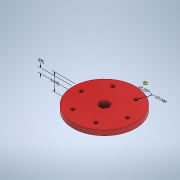
# Autodesk Inventor part: attachementToTripod
Saved by Autodesk Inventor 2022 (Build 260153000, 153)
## iProperties
Created: 2021-02-15
Part Number: attachementToTripod
Material: PC/ABS Plastic
Document SubType Name: Modeling
Designer: robst
Density: 0.357273 g/cm^3
Appearance: Red
Author: robst
Autodesk Inventor part; units mm, degrees
ref_plane "YZ Plane" through (0, 0, 0) normal (1, 0, 0) x (0, 1, 0)
ref_plane "XZ Plane" through (0, 0, 0) normal (0, 1, 0) x (-1, 0, 0)
ref_plane "XY Plane" through (0, 0, 0) normal (0, 0, 1) x (1, 0, 0)
sketch "Sketch2" plane through (0, 0, 0) normal (0, 0, 1) x (1, 0, 0)
  line L0 (-60.325, 0) -> (-60.325, -9.525)
  line L1 (-60.325, -9.525) -> (-12.7, -9.525)
  line L2 (-10.795, -44.525) -> (0, -44.525)
  line L3 (-60.325, 0) -> (0, 0)
  line L4 (0, 0) -> (0, -44.525) construction
  line L5 (0, 0) -> (0, -44.525)
  line L6 (0, -53.43) -> (0, 8.905) projected
  line L7 (-12.7, -9.525) -> (-10.795, -44.525)
  dimension "d0" = 60.325
  dimension "d3" = 9.525
  dimension "d4" = 35
  dimension "d64" = 10.795
  constraints: 14 end point, 3 vertical, 2 horizontal, 1 perpendicular
  measures "d0" distance from line of L0 L3.end
  measures "d3" distance from line of L1 L3.end
  measures "d4" distance from line of L2.start L1
  measures "d64" horizontal distance of L2.start L3.end
revolve "Revolution1" add sketch "Sketch2" angle 360 about axis through (0, -10, 0) along (0, 1, 0)
sketch "Sketch5" plane through (0, -9.525, 0) normal (0, -1, 0) x (1, 0, 0)
  circle A0 centre (0, 0) radius 34.925 construction
  line L0 (30.2767, -23.2881) -> (30.3048, -23.2474)
  spline S0 degree 2 poles (30.3048, -23.2474) (30.4192, -23.1689) (30.7643, -22.822) (30.8732, -22.6645) knots 0 0 0 1 2 2 2
  spline S1 degree 2 poles (30.8732, -22.6645) (31.2175, -22.1669) (31.0657, -21.4311) (30.4766, -21.0236) knots 0 0 0 1 2 2 2
  line L1 (30.4766, -21.0236) -> (30.3192, -20.9147)
  line L2 (30.3192, -20.9147) -> (29.4128, -22.2249)
  line L3 (29.4128, -22.2249) -> (28.7577, -21.7717)
  line L4 (28.7577, -21.7717) -> (29.6465, -20.4869)
  line L5 (29.6465, -20.4869) -> (25.5991, -17.6869)
  line L6 (25.5991, -17.6869) -> (26.1472, -16.8947)
  line L7 (26.1472, -16.8947) -> (30.1946, -19.6947)
  line L8 (30.1946, -19.6947) -> (30.5635, -19.1615)
  line L9 (30.5635, -19.1615) -> (31.2186, -19.6147)
  line L10 (31.2186, -19.6147) -> (30.8497, -20.1479)
  line L11 (30.8497, -20.1479) -> (31.0071, -20.2568)
  spline S2 degree 2 poles (31.0071, -20.2568) (31.8501, -20.84) (32.1681, -22.2689) (31.6411, -23.0306) knots 0 0 0 1 2 2 2
  spline S3 degree 2 poles (31.6411, -23.0306) (31.4901, -23.249) (31.1528, -23.6389) (31.0029, -23.7904) knots 0 0 0 1 2 2 2
  line L12 (31.0029, -23.7904) -> (30.2767, -23.2881)
  line L13 (23.4719, -20.4315) -> (24.0931, -19.6952)
  line L14 (24.0931, -19.6952) -> (28.4636, -23.3822)
  line L15 (28.4636, -23.3822) -> (27.8425, -24.1185)
  line L16 (27.8425, -24.1185) -> (23.4719, -20.4315)
  line L17 (28.5256, -24.7836) -> (29.2303, -23.9482)
  line L18 (29.2303, -23.9482) -> (29.9949, -24.5933)
  line L19 (29.9949, -24.5933) -> (29.2902, -25.4287)
  line L20 (29.2902, -25.4287) -> (28.5256, -24.7836)
  line L21 (21.8315, -22.1757) -> (22.5074, -21.4893)
  line L22 (22.5074, -21.4893) -> (28.1787, -27.0744)
  line L23 (28.1787, -27.0744) -> (27.5027, -27.7607)
  line L24 (27.5027, -27.7607) -> (21.8315, -22.1757)
  spline S4 degree 2 poles (18.8163, -24.6214) (19.8941, -23.7743) (22.0288, -24.0519) (22.9065, -25.1685) knots 0 0 0 1 2 2 2
  spline S5 degree 2 poles (22.9065, -25.1685) (23.769, -26.2657) (23.6412, -28.4712) (22.7139, -29.2001) knots 0 0 0 1 2 2 2
  spline S6 degree 2 poles (22.7139, -29.2001) (22.2964, -29.5282) (21.4599, -29.7931) (21.0198, -29.7227) knots 0 0 0 1 2 2 2
  spline S7 degree 2 poles (21.0198, -29.7227) (20.5748, -29.6563) (19.7336, -29.1157) (19.31, -28.5769) knots 0 0 0 1 2 2 2
  line L25 (19.31, -28.5769) -> (18.9857, -28.1642)
  line L26 (18.9857, -28.1642) -> (22.0975, -25.7181)
  spline S8 degree 2 poles (22.0975, -25.7181) (21.4831, -24.9365) (20.0441, -24.7245) (19.345, -25.2741) knots 0 0 0 1 2 2 2
  spline S9 degree 2 poles (19.345, -25.2741) (19.0974, -25.4687) (18.7046, -25.9581) (18.5791, -26.1982) knots 0 0 0 1 2 2 2
  spline S10 degree 2 poles (18.5791, -26.1982) (18.4515, -26.4555) (18.3035, -26.8468) (18.2723, -26.997) knots 0 0 0 1 2 2 2
  line L27 (18.2723, -26.997) -> (18.2286, -27.0313)
  line L28 (18.2286, -27.0313) -> (17.5799, -26.206)
  spline S11 degree 2 poles (17.5799, -26.206) (17.669, -26.0496) (17.945, -25.5813) (18.066, -25.4155) knots 0 0 0 1 2 2 2
  spline S12 degree 2 poles (18.066, -25.4155) (18.2348, -25.1807) (18.5444, -24.8352) (18.8163, -24.6214) knots 0 0 0 1 2 2 2
  spline S13 degree 2 poles (20.1777, -28.1619) (20.4278, -28.4601) (20.9051, -28.8075) (21.1448, -28.8626) knots 0 0 0 1 2 2 2
  spline S14 degree 2 poles (21.1448, -28.8626) (21.4094, -28.9295) (21.9633, -28.7847) (22.2691, -28.5443) knots 0 0 0 1 2 2 2
  spline S15 degree 2 poles (22.2691, -28.5443) (22.5701, -28.3077) (22.8513, -27.7961) (22.8887, -27.4839) knots 0 0 0 1 2 2 2
  spline S16 degree 2 poles (22.8887, -27.4839) (22.9174, -27.1707) (22.7525, -26.6013) (22.5516, -26.2958) knots 0 0 0 1 2 2 2
  line L29 (22.5516, -26.2958) -> (20.1777, -28.1619)
  line L30 (16.9957, -31.0317) -> (18.0577, -30.426)
  line L31 (18.0577, -30.426) -> (18.7797, -31.6918)
  line L32 (18.7797, -31.6918) -> (17.7177, -32.2976)
  line L33 (17.7177, -32.2976) -> (16.9957, -31.0317)
  line L34 (14.8847, -27.3306) -> (15.9467, -26.7249)
  line L35 (15.9467, -26.7249) -> (16.6687, -27.9907)
  line L36 (16.6687, -27.9907) -> (15.6067, -28.5965)
  line L37 (15.6067, -28.5965) -> (14.8847, -27.3306)
  spline S17 degree 2 poles (7.233, -30.9053) (7.3235, -30.7911) (7.6238, -30.3894) (7.7783, -30.2514) knots 0 0 0 1 2 2 2
  spline S18 degree 2 poles (7.7783, -30.2514) (7.9869, -30.0538) (8.4084, -29.792) (8.8255, -29.6785) knots 0 0 0 1 2 2 2
  spline S19 degree 2 poles (8.8255, -29.6785) (9.1652, -29.5861) (9.8486, -29.6754) (10.1442, -29.8446) knots 0 0 0 1 2 2 2
  spline S20 degree 2 poles (10.1442, -29.8446) (10.4262, -30.011) (10.8759, -30.6054) (10.9764, -30.9748) knots 0 0 0 1 2 2 2
  spline S21 degree 2 poles (10.9764, -30.9748) (11.132, -31.5469) (10.8698, -32.4885) (10.4087, -32.8635) knots 0 0 0 1 2 2 2
  spline S22 degree 2 poles (10.4087, -32.8635) (10.0023, -33.2045) (8.7828, -33.709) (8.0613, -33.9501) knots 0 0 0 1 2 2 2
  line L38 (8.0613, -33.9501) -> (8.1099, -34.1288)
  spline S23 degree 2 poles (8.1099, -34.1288) (8.1974, -34.4506) (8.5027, -34.7963) (8.7122, -34.8609) knots 0 0 0 1 2 2 2
  spline S24 degree 2 poles (8.7122, -34.8609) (8.9218, -34.9255) (9.4537, -34.8576) (9.7278, -34.783) knots 0 0 0 1 2 2 2
  spline S25 degree 2 poles (9.7278, -34.783) (10.0495, -34.6955) (10.8676, -34.2682) (11.2523, -33.9651) knots 0 0 0 1 2 2 2
  line L39 (11.2523, -33.9651) -> (11.3059, -33.9505)
  line L40 (11.3059, -33.9505) -> (11.5637, -34.8979)
  spline S26 degree 2 poles (11.5637, -34.8979) (11.3269, -35.0391) (10.4162, -35.4789) (9.9455, -35.6069) knots 0 0 0 1 2 2 2
  spline S27 degree 2 poles (9.9455, -35.6069) (9.3735, -35.7625) (8.5443, -35.7961) (8.1712, -35.648) knots 0 0 0 1 2 2 2
  spline S28 degree 2 poles (8.1712, -35.648) (7.8057, -35.5043) (7.3117, -34.8643) (7.1707, -34.3459) knots 0 0 0 1 2 2 2
  line L41 (7.1707, -34.3459) -> (6.1446, -30.5742)
  line L42 (6.1446, -30.5742) -> (7.0742, -30.3213)
  line L43 (7.0742, -30.3213) -> (7.233, -30.9053)
  line L44 (7.4437, -31.6799) -> (7.8603, -33.2112)
  spline S29 degree 2 poles (7.8603, -33.2112) (8.1859, -33.0906) (9.1653, -32.7154) (9.4552, -32.5342) knots 0 0 0 1 2 2 2
  spline S30 degree 2 poles (9.4552, -32.5342) (9.7938, -32.3205) (10.1484, -31.7184) (10.0349, -31.3014) knots 0 0 0 1 2 2 2
  spline S31 degree 2 poles (10.0349, -31.3014) (9.9052, -30.8247) (9.2377, -30.4879) (8.7253, -30.6273) knots 0 0 0 1 2 2 2
  spline S32 degree 2 poles (8.7253, -30.6273) (8.2903, -30.7456) (7.6774, -31.3155) (7.4437, -31.6799) knots 0 0 0 1 2 2 2
  spline S33 degree 2 poles (3.0779, -30.858) (3.8564, -30.7633) (4.8411, -31.5454) (4.9582, -32.5078) knots 0 0 0 1 2 2 2
  line L45 (4.9582, -32.5078) -> (5.341, -35.6524)
  line L46 (5.341, -35.6524) -> (5.9846, -35.574)
  line L47 (5.9846, -35.574) -> (6.0809, -36.3648)
  line L48 (6.0809, -36.3648) -> (5.4372, -36.4431)
  line L49 (5.4372, -36.4431) -> (5.6357, -38.0737)
  line L50 (5.6357, -38.0737) -> (4.6794, -38.19)
  line L51 (4.6794, -38.19) -> (4.481, -36.5595)
  line L52 (4.481, -36.5595) -> (2.7217, -36.7736)
  line L53 (2.7217, -36.7736) -> (2.6255, -35.9829)
  line L54 (2.6255, -35.9829) -> (4.3847, -35.7688)
  line L55 (4.3847, -35.7688) -> (4.0557, -33.0655)
  spline S34 degree 2 poles (4.0557, -33.0655) (4.0035, -32.6364) (3.9154, -32.1682) (3.7866, -31.9786) knots 0 0 0 1 2 2 2
  spline S35 degree 2 poles (3.7866, -31.9786) (3.6791, -31.8113) (3.2713, -31.6805) (2.9403, -31.7208) knots 0 0 0 1 2 2 2
  spline S36 degree 2 poles (2.9403, -31.7208) (2.7073, -31.7491) (2.2893, -31.9431) (2.1964, -31.9979) knots 0 0 0 1 2 2 2
  line L56 (2.1964, -31.9979) -> (2.1413, -32.0047)
  line L57 (2.1413, -32.0047) -> (2.0368, -31.1465)
  spline S37 degree 2 poles (2.0368, -31.1465) (2.2976, -31.0401) (2.8388, -30.8871) (3.0779, -30.858) knots 0 0 0 1 2 2 2
  spline S38 degree 2 poles (-0.4091, -31.0085) (0.3751, -31.0018) (1.2658, -31.8896) (1.274, -32.8591) knots 0 0 0 1 2 2 2
  line L58 (1.274, -32.8591) -> (1.301, -36.0267)
  line L59 (1.301, -36.0267) -> (1.9493, -36.0212)
  line L60 (1.9493, -36.0212) -> (1.9561, -36.8178)
  line L61 (1.9561, -36.8178) -> (1.3078, -36.8233)
  line L62 (1.3078, -36.8233) -> (1.3218, -38.4658)
  line L63 (1.3218, -38.4658) -> (0.3585, -38.474)
  line L64 (0.3585, -38.474) -> (0.3445, -36.8315)
  line L65 (0.3445, -36.8315) -> (-1.4277, -36.8466)
  line L66 (-1.4277, -36.8466) -> (-1.4344, -36.05)
  line L67 (-1.4344, -36.05) -> (0.3377, -36.0349)
  line L68 (0.3377, -36.0349) -> (0.3145, -33.3118)
  spline S39 degree 2 poles (0.3145, -33.3118) (0.3109, -32.8796) (0.2759, -32.4044) (0.1692, -32.2015) knots 0 0 0 1 2 2 2
  spline S40 degree 2 poles (0.1692, -32.2015) (0.0813, -32.0232) (-0.3093, -31.8474) (-0.6427, -31.8503) knots 0 0 0 1 2 2 2
  spline S41 degree 2 poles (-0.6427, -31.8503) (-0.8774, -31.8523) (-1.3146, -31.998) (-1.413, -32.0421) knots 0 0 0 1 2 2 2
  line L69 (-1.413, -32.0421) -> (-1.4686, -32.0426)
  line L70 (-1.4686, -32.0426) -> (-1.4759, -31.1781)
  spline S42 degree 2 poles (-1.4759, -31.1781) (-1.2049, -31.1017) (-0.6499, -31.0105) (-0.4091, -31.0085) knots 0 0 0 1 2 2 2
  spline S43 degree 2 poles (-5.4224, -31.2738) (-5.2945, -31.204) (-4.8611, -30.9517) (-4.665, -30.885) knots 0 0 0 1 2 2 2
  spline S44 degree 2 poles (-4.665, -30.885) (-4.3957, -30.7848) (-3.9054, -30.7085) (-3.4771, -30.7671) knots 0 0 0 1 2 2 2
  spline S45 degree 2 poles (-3.4771, -30.7671) (-3.1284, -30.8148) (-2.5342, -31.1641) (-2.3282, -31.4353) knots 0 0 0 1 2 2 2
  spline S46 degree 2 poles (-2.3282, -31.4353) (-2.1337, -31.6988) (-1.9521, -32.4217) (-2.004, -32.801) knots 0 0 0 1 2 2 2
  spline S47 degree 2 poles (-2.004, -32.801) (-2.0844, -33.3883) (-2.6938, -34.1526) (-3.2648, -34.3175) knots 0 0 0 1 2 2 2
  spline S48 degree 2 poles (-3.2648, -34.3175) (-3.7722, -34.4725) (-5.0918, -34.4602) (-5.8502, -34.4001) knots 0 0 0 1 2 2 2
  line L71 (-5.8502, -34.4001) -> (-5.8753, -34.5836)
  spline S49 degree 2 poles (-5.8753, -34.5836) (-5.9205, -34.914) (-5.7747, -35.3516) (-5.607, -35.4929) knots 0 0 0 1 2 2 2
  spline S50 degree 2 poles (-5.607, -35.4929) (-5.4394, -35.6343) (-4.9233, -35.7797) (-4.6418, -35.8182) knots 0 0 0 1 2 2 2
  spline S51 degree 2 poles (-4.6418, -35.8182) (-4.3115, -35.8634) (-3.3914, -35.7898) (-2.9189, -35.6612) knots 0 0 0 1 2 2 2
  line L72 (-2.9189, -35.6612) -> (-2.8638, -35.6688)
  line L73 (-2.8638, -35.6688) -> (-2.9969, -36.6415)
  spline S52 degree 2 poles (-2.9969, -36.6415) (-3.27, -36.679) (-4.2801, -36.7277) (-4.7635, -36.6616) knots 0 0 0 1 2 2 2
  spline S53 degree 2 poles (-4.7635, -36.6616) (-5.3508, -36.5813) (-6.1272, -36.2881) (-6.4127, -36.0059) knots 0 0 0 1 2 2 2
  spline S54 degree 2 poles (-6.4127, -36.0059) (-6.6929, -35.7308) (-6.8975, -34.9486) (-6.8247, -34.4164) knots 0 0 0 1 2 2 2
  line L74 (-6.8247, -34.4164) -> (-6.2948, -30.5436)
  line L75 (-6.2948, -30.5436) -> (-5.3404, -30.6742)
  line L76 (-5.3404, -30.6742) -> (-5.4224, -31.2738)
  line L77 (-5.5312, -32.0691) -> (-5.7464, -33.6415)
  spline S55 degree 2 poles (-5.7464, -33.6415) (-5.3996, -33.6577) (-4.3514, -33.6952) (-4.0137, -33.6417) knots 0 0 0 1 2 2 2
  spline S56 degree 2 poles (-4.0137, -33.6417) (-3.6185, -33.5773) (-3.0568, -33.1618) (-2.9982, -32.7335) knots 0 0 0 1 2 2 2
  spline S57 degree 2 poles (-2.9982, -32.7335) (-2.9313, -32.2441) (-3.4141, -31.6732) (-3.9402, -31.6012) knots 0 0 0 1 2 2 2
  spline S58 degree 2 poles (-3.9402, -31.6012) (-4.3869, -31.5401) (-5.1738, -31.8251) (-5.5312, -32.0691) knots 0 0 0 1 2 2 2
  spline S59 degree 2 poles (-9.7347, -29.4216) (-9.1687, -29.5978) (-8.3394, -30.2374) (-8.1135, -30.6957) knots 0 0 0 1 2 2 2
  spline S60 degree 2 poles (-8.1135, -30.6957) (-7.8856, -31.1482) (-7.8481, -32.3369) (-8.072, -33.0562) knots 0 0 0 1 2 2 2
  spline S61 degree 2 poles (-8.072, -33.0562) (-8.2958, -33.7755) (-9.0057, -34.7058) (-9.4401, -34.9586) knots 0 0 0 1 2 2 2
  spline S62 degree 2 poles (-9.4401, -34.9586) (-9.8763, -35.2174) (-10.9566, -35.3016) (-11.5108, -35.1291) knots 0 0 0 1 2 2 2
  spline S63 degree 2 poles (-11.5108, -35.1291) (-11.9589, -34.9896) (-12.7173, -34.4755) (-12.9902, -34.2095) knots 0 0 0 1 2 2 2
  line L78 (-12.9902, -34.2095) -> (-12.6691, -33.1777)
  line L79 (-12.6691, -33.1777) -> (-12.616, -33.1942)
  spline S64 degree 2 poles (-12.616, -33.1942) (-12.5415, -33.308) (-12.301, -33.6156) (-12.1177, -33.7956) knots 0 0 0 1 2 2 2
  spline S65 degree 2 poles (-12.1177, -33.7956) (-11.9524, -33.9504) (-11.4795, -34.2593) (-11.2436, -34.3327) knots 0 0 0 1 2 2 2
  spline S66 degree 2 poles (-11.2436, -34.3327) (-10.5302, -34.5547) (-9.3277, -33.7455) (-9.0212, -32.7608) knots 0 0 0 1 2 2 2
  spline S67 degree 2 poles (-9.0212, -32.7608) (-8.7222, -31.7997) (-9.2236, -30.4602) (-9.9666, -30.229) knots 0 0 0 1 2 2 2
  spline S68 degree 2 poles (-9.9666, -30.229) (-10.4147, -30.0895) (-11.3439, -30.2078) (-11.7463, -30.3995) knots 0 0 0 1 2 2 2
  line L80 (-11.7463, -30.3995) -> (-11.7994, -30.3829)
  line L81 (-11.7994, -30.3829) -> (-11.4783, -29.3511)
  spline S69 degree 2 poles (-11.4783, -29.3511) (-11.3225, -29.3285) (-10.8529, -29.2741) (-10.6749, -29.2842) knots 0 0 0 1 2 2 2
  spline S70 degree 2 poles (-10.6749, -29.2842) (-10.4171, -29.2869) (-10.0236, -29.3317) (-9.7347, -29.4216) knots 0 0 0 1 2 2 2
  line L82 (-16.1877, -26.669) -> (-15.3301, -27.1077)
  line L83 (-15.3301, -27.1077) -> (-16.8149, -30.0104)
  spline S71 degree 2 poles (-16.8149, -30.0104) (-16.9949, -30.3623) (-17.2383, -31.0007) (-17.2321, -31.2328) knots 0 0 0 1 2 2 2
  spline S72 degree 2 poles (-17.2321, -31.2328) (-17.2261, -31.4786) (-16.9479, -31.8568) (-16.629, -32.0199) knots 0 0 0 1 2 2 2
  spline S73 degree 2 poles (-16.629, -32.0199) (-16.3102, -32.183) (-15.4596, -32.188) (-14.9947, -32.0791) knots 0 0 0 1 2 2 2
  line L84 (-14.9947, -32.0791) -> (-13.0486, -28.2748)
  line L85 (-13.0486, -28.2748) -> (-12.191, -28.7135)
  line L86 (-12.191, -28.7135) -> (-15.8159, -35.7998)
  line L87 (-15.8159, -35.7998) -> (-16.6735, -35.3611)
  line L88 (-16.6735, -35.3611) -> (-15.363, -32.7992)
  spline S74 degree 2 poles (-15.363, -32.7992) (-15.925, -32.9487) (-16.8528, -32.9319) (-17.2706, -32.7182) knots 0 0 0 1 2 2 2
  spline S75 degree 2 poles (-17.2706, -32.7182) (-18.0183, -32.3357) (-18.3587, -30.9131) (-17.8778, -29.973) knots 0 0 0 1 2 2 2
  line L89 (-17.8778, -29.973) -> (-16.1877, -26.669)
  spline S76 degree 2 poles (-19.2059, -24.3188) (-18.1186, -25.1537) (-17.8599, -27.2908) (-18.7248, -28.4173) knots 0 0 0 1 2 2 2
  spline S77 degree 2 poles (-18.7248, -28.4173) (-19.5747, -29.5242) (-21.7434, -29.9456) (-22.6789, -29.2273) knots 0 0 0 1 2 2 2
  spline S78 degree 2 poles (-22.6789, -29.2273) (-23.1001, -28.9039) (-23.5635, -28.1588) (-23.6041, -27.7149) knots 0 0 0 1 2 2 2
  spline S79 degree 2 poles (-23.6041, -27.7149) (-23.6497, -27.2673) (-23.3339, -26.3186) (-22.9165, -25.775) knots 0 0 0 1 2 2 2
  line L90 (-22.9165, -25.775) -> (-22.5968, -25.3587)
  line L91 (-22.5968, -25.3587) -> (-19.4573, -27.7693)
  spline S80 degree 2 poles (-19.4573, -27.7693) (-18.8519, -26.9807) (-19.0022, -25.534) (-19.7075, -24.9924) knots 0 0 0 1 2 2 2
  spline S81 degree 2 poles (-19.7075, -24.9924) (-19.9573, -24.8006) (-20.5287, -24.541) (-20.7923, -24.4787) knots 0 0 0 1 2 2 2
  spline S82 degree 2 poles (-20.7923, -24.4787) (-21.0732, -24.4187) (-21.4889, -24.372) (-21.6421, -24.3789) knots 0 0 0 1 2 2 2
  line L92 (-21.6421, -24.3789) -> (-21.6862, -24.3451)
  line L93 (-21.6862, -24.3451) -> (-21.0469, -23.5125)
  spline S83 degree 2 poles (-21.0469, -23.5125) (-20.8733, -23.5601) (-20.3513, -23.7118) (-20.1608, -23.788) knots 0 0 0 1 2 2 2
  spline S84 degree 2 poles (-20.1608, -23.788) (-19.8915, -23.8936) (-19.4801, -24.1082) (-19.2059, -24.3188) knots 0 0 0 1 2 2 2
  spline S85 degree 2 poles (-22.2999, -26.5131) (-22.527, -26.8292) (-22.7456, -27.3776) (-22.7398, -27.6234) knots 0 0 0 1 2 2 2
  spline S86 degree 2 poles (-22.7398, -27.6234) (-22.7392, -27.8964) (-22.462, -28.3973) (-22.1534, -28.6342) knots 0 0 0 1 2 2 2
  spline S87 degree 2 poles (-22.1534, -28.6342) (-21.8498, -28.8674) (-21.2845, -29.0133) (-20.9728, -28.9724) knots 0 0 0 1 2 2 2
  spline S88 degree 2 poles (-20.9728, -28.9724) (-20.6622, -28.9228) (-20.1512, -28.6223) (-19.9048, -28.3521) knots 0 0 0 1 2 2 2
  line L94 (-19.9048, -28.3521) -> (-22.2999, -26.5131)
  line L95 (-25.8186, -17.5864) -> (-28.3773, -19.6859)
  spline S89 degree 2 poles (-28.3773, -19.6859) (-28.6828, -19.9366) (-29.164, -20.4113) (-29.2445, -20.6052) knots 0 0 0 1 2 2 2
  spline S90 degree 2 poles (-29.2445, -20.6052) (-29.3394, -20.8108) (-29.2532, -21.2274) (-29.0456, -21.4804) knots 0 0 0 1 2 2 2
  spline S91 degree 2 poles (-29.0456, -21.4804) (-28.8576, -21.7095) (-28.1451, -22.0035) (-27.6506, -22.061) knots 0 0 0 1 2 2 2
  spline S92 degree 2 poles (-27.6506, -22.061) (-27.5877, -22.0014) (-27.4093, -21.8391) (-27.2852, -21.7373) knots 0 0 0 1 2 2 2
  line L96 (-27.2852, -21.7373) -> (-24.3732, -19.3479)
  line L97 (-24.3732, -19.3479) -> (-23.7622, -20.0926)
  line L98 (-23.7622, -20.0926) -> (-26.3209, -22.1921)
  spline S93 degree 2 poles (-26.3209, -22.1921) (-26.6264, -22.4428) (-27.1076, -22.9175) (-27.1881, -23.1114) knots 0 0 0 1 2 2 2
  spline S94 degree 2 poles (-27.1881, -23.1114) (-27.283, -23.317) (-27.1968, -23.7336) (-26.9892, -23.9866) knots 0 0 0 1 2 2 2
  spline S95 degree 2 poles (-26.9892, -23.9866) (-26.7934, -24.2253) (-26.0578, -24.5084) (-25.6202, -24.5647) knots 0 0 0 1 2 2 2
  line L99 (-25.6202, -24.5647) -> (-22.3168, -21.8541)
  line L100 (-22.3168, -21.8541) -> (-21.7058, -22.5988)
  line L101 (-21.7058, -22.5988) -> (-26.1262, -26.2259)
  line L102 (-26.1262, -26.2259) -> (-26.7373, -25.4812)
  line L103 (-26.7373, -25.4812) -> (-26.2504, -25.0817)
  spline S96 degree 2 poles (-26.2504, -25.0817) (-26.7805, -25.0295) (-27.5704, -24.719) (-27.8524, -24.3753) knots 0 0 0 1 2 2 2
  spline S97 degree 2 poles (-27.8524, -24.3753) (-28.1736, -23.9839) (-28.313, -23.0839) (-28.0365, -22.5934) knots 0 0 0 1 2 2 2
  spline S98 degree 2 poles (-28.0365, -22.5934) (-28.6917, -22.5639) (-29.6033, -22.2415) (-29.9088, -21.8691) knots 0 0 0 1 2 2 2
  spline S99 degree 2 poles (-29.9088, -21.8691) (-30.1438, -21.5827) (-30.3511, -20.97) (-30.2916, -20.6336) knots 0 0 0 1 2 2 2
  spline S100 degree 2 poles (-30.2916, -20.6336) (-30.236, -20.2924) (-29.7951, -19.6032) (-29.3416, -19.2311) knots 0 0 0 1 2 2 2
  line L104 (-29.3416, -19.2311) -> (-26.4296, -16.8417)
  line L105 (-26.4296, -16.8417) -> (-25.8186, -17.5864)
  spline S101 degree 2 poles (-27.9752, -13.3288) (-27.3687, -14.5582) (-28.0811, -16.5897) (-29.3548, -17.218) knots 0 0 0 1 2 2 2
  spline S102 degree 2 poles (-29.3548, -17.218) (-30.6063, -17.8354) (-32.7379, -17.2551) (-33.2597, -16.1974) knots 0 0 0 1 2 2 2
  spline S103 degree 2 poles (-33.2597, -16.1974) (-33.4947, -15.7211) (-33.5811, -14.848) (-33.4215, -14.4318) knots 0 0 0 1 2 2 2
  spline S104 degree 2 poles (-33.4215, -14.4318) (-33.2646, -14.0102) (-32.5621, -13.2987) (-31.9474, -12.9954) knots 0 0 0 1 2 2 2
  line L106 (-31.9474, -12.9954) -> (-31.4766, -12.7632)
  line L107 (-31.4766, -12.7632) -> (-29.7255, -16.313)
  spline S105 degree 2 poles (-29.7255, -16.313) (-28.8339, -15.8732) (-28.3295, -14.5089) (-28.7229, -13.7114) knots 0 0 0 1 2 2 2
  spline S106 degree 2 poles (-28.7229, -13.7114) (-28.8622, -13.429) (-29.26, -12.9436) (-29.469, -12.7712) knots 0 0 0 1 2 2 2
  spline S107 degree 2 poles (-29.469, -12.7712) (-29.6945, -12.5933) (-30.0468, -12.3677) (-30.1873, -12.3062) knots 0 0 0 1 2 2 2
  line L108 (-30.1873, -12.3062) -> (-30.2119, -12.2564)
  line L109 (-30.2119, -12.2564) -> (-29.2704, -11.7919)
  spline S108 degree 2 poles (-29.2704, -11.7919) (-29.1358, -11.9114) (-28.7345, -12.2781) (-28.5973, -12.4307) knots 0 0 0 1 2 2 2
  spline S109 degree 2 poles (-28.5973, -12.4307) (-28.4023, -12.6444) (-28.1282, -13.0187) (-27.9752, -13.3288) knots 0 0 0 1 2 2 2
  spline S110 degree 2 poles (-31.7204, -13.9301) (-32.0638, -14.1133) (-32.5023, -14.5086) (-32.6057, -14.7317) knots 0 0 0 1 2 2 2
  spline S111 degree 2 poles (-32.6057, -14.7317) (-32.7257, -14.9769) (-32.6984, -15.5486) (-32.5263, -15.8975) knots 0 0 0 1 2 2 2
  spline S112 degree 2 poles (-32.5263, -15.8975) (-32.3569, -16.2409) (-31.9143, -16.6216) (-31.6166, -16.7226) knots 0 0 0 1 2 2 2
  spline S113 degree 2 poles (-31.6166, -16.7226) (-31.3161, -16.8154) (-30.7249, -16.7716) (-30.3845, -16.6381) knots 0 0 0 1 2 2 2
  line L110 (-30.3845, -16.6381) -> (-31.7204, -13.9301)
  line L111 (-30.553, -6.308) -> (-30.2903, -7.2347)
  line L112 (-30.2903, -7.2347) -> (-33.427, -8.1242)
  spline S114 degree 2 poles (-33.427, -8.1242) (-33.8072, -8.232) (-34.4405, -8.4886) (-34.6062, -8.6511) knots 0 0 0 1 2 2 2
  spline S115 degree 2 poles (-34.6062, -8.6511) (-34.7821, -8.8229) (-34.8696, -9.2842) (-34.7719, -9.6288) knots 0 0 0 1 2 2 2
  spline S116 degree 2 poles (-34.7719, -9.6288) (-34.6742, -9.9733) (-34.0986, -10.5996) (-33.7022, -10.8659) knots 0 0 0 1 2 2 2
  line L113 (-33.7022, -10.8659) -> (-29.5912, -9.7002)
  line L114 (-29.5912, -9.7002) -> (-29.3284, -10.6269)
  line L115 (-29.3284, -10.6269) -> (-34.8296, -12.1868)
  line L116 (-34.8296, -12.1868) -> (-35.0924, -11.2601)
  line L117 (-35.0924, -11.2601) -> (-34.4805, -11.0866)
  spline S117 degree 2 poles (-34.4805, -11.0866) (-34.9727, -10.7768) (-35.5922, -10.086) (-35.7202, -9.6345) knots 0 0 0 1 2 2 2
  spline S118 degree 2 poles (-35.7202, -9.6345) (-35.9493, -8.8265) (-35.1394, -7.6084) (-34.1235, -7.3204) knots 0 0 0 1 2 2 2
  line L118 (-34.1235, -7.3204) -> (-30.553, -6.308)
  spline S119 degree 2 poles (-30.8413, -3.2409) (-30.7425, -4.0189) (-31.5194, -5.0077) (-32.4811, -5.13) knots 0 0 0 1 2 2 2
  line L119 (-32.4811, -5.13) -> (-35.6237, -5.5293)
  line L120 (-35.6237, -5.5293) -> (-35.5419, -6.1725)
  line L121 (-35.5419, -6.1725) -> (-36.3321, -6.273)
  line L122 (-36.3321, -6.273) -> (-36.4139, -5.6297)
  line L123 (-36.4139, -5.6297) -> (-38.0433, -5.8368)
  line L124 (-38.0433, -5.8368) -> (-38.1648, -4.8812)
  line L125 (-38.1648, -4.8812) -> (-36.5353, -4.6741)
  line L126 (-36.5353, -4.6741) -> (-36.7587, -2.916)
  line L127 (-36.7587, -2.916) -> (-35.9685, -2.8156)
  line L128 (-35.9685, -2.8156) -> (-35.7451, -4.5737)
  line L129 (-35.7451, -4.5737) -> (-33.0436, -4.2304)
  spline S120 degree 2 poles (-33.0436, -4.2304) (-32.6148, -4.1759) (-32.147, -4.0853) (-31.9581, -3.9555) knots 0 0 0 1 2 2 2
  spline S121 degree 2 poles (-31.9581, -3.9555) (-31.7914, -3.8472) (-31.6628, -3.4387) (-31.7048, -3.1079) knots 0 0 0 1 2 2 2
  spline S122 degree 2 poles (-31.7048, -3.1079) (-31.7344, -2.8751) (-31.9306, -2.4581) (-31.9859, -2.3655) knots 0 0 0 1 2 2 2
  line L130 (-31.9859, -2.3655) -> (-31.9929, -2.3104)
  line L131 (-31.9929, -2.3104) -> (-31.1353, -2.2014)
  spline S123 degree 2 poles (-31.1353, -2.2014) (-31.0275, -2.4616) (-30.8717, -3.002) (-30.8413, -3.2409) knots 0 0 0 1 2 2 2
  line L132 (-31.1171, 0.3593) -> (-37.833, 0.5475)
  line L133 (-37.833, 0.5475) -> (-37.9046, -2.0079)
  line L134 (-37.9046, -2.0079) -> (-38.8058, -1.9827)
  line L135 (-38.8058, -1.9827) -> (-38.6342, 4.1405)
  line L136 (-38.6342, 4.1405) -> (-37.733, 4.1153)
  line L137 (-37.733, 4.1153) -> (-37.8046, 1.5598)
  line L138 (-37.8046, 1.5598) -> (-31.0888, 1.3716)
  line L139 (-31.0888, 1.3716) -> (-31.1171, 0.3593)
  spline S124 degree 2 poles (-32.6248, 9.8171) (-31.2139, 9.5056) (-29.9758, 7.8094) (-30.226, 6.6758) knots 0 0 0 1 2 2 2
  spline S125 degree 2 poles (-30.226, 6.6758) (-30.4829, 5.512) (-32.363, 4.5295) (-33.7257, 4.8304) knots 0 0 0 1 2 2 2
  spline S126 degree 2 poles (-33.7257, 4.8304) (-35.1246, 5.1392) (-36.3708, 6.8561) (-36.1232, 7.9777) knots 0 0 0 1 2 2 2
  spline S127 degree 2 poles (-36.1232, 7.9777) (-35.873, 9.1113) (-34.0298, 10.1272) (-32.6248, 9.8171) knots 0 0 0 1 2 2 2
  spline S128 degree 2 poles (-32.8392, 8.8463) (-33.9245, 9.0859) (-35.1541, 8.5289) (-35.3152, 7.7993) knots 0 0 0 1 2 2 2
  spline S129 degree 2 poles (-35.3152, 7.7993) (-35.4763, 7.0697) (-34.5968, 6.0408) (-33.5114, 5.8012) knots 0 0 0 1 2 2 2
  spline S130 degree 2 poles (-33.5114, 5.8012) (-32.4562, 5.5682) (-31.1951, 6.1246) (-31.034, 6.8542) knots 0 0 0 1 2 2 2
  spline S131 degree 2 poles (-31.034, 6.8542) (-30.8743, 7.5778) (-31.7658, 8.6093) (-32.8392, 8.8463) knots 0 0 0 1 2 2 2
  line L140 (-28.7817, 11.8329) -> (-34.9526, 14.4895)
  line L141 (-34.9526, 14.4895) -> (-35.9635, 12.1414)
  line L142 (-35.9635, 12.1414) -> (-36.7916, 12.4979)
  line L143 (-36.7916, 12.4979) -> (-34.3694, 18.1243)
  line L144 (-34.3694, 18.1243) -> (-33.5413, 17.7678)
  line L145 (-33.5413, 17.7678) -> (-34.5522, 15.4197)
  line L146 (-34.5522, 15.4197) -> (-28.3813, 12.763)
  line L147 (-28.3813, 12.763) -> (-28.7817, 11.8329)
  line L148 (-29.2463, 20.7319) -> (-29.2728, 20.6902)
  spline S132 degree 2 poles (-29.2728, 20.6902) (-29.3584, 20.6129) (-29.4978, 20.4161) (-29.5871, 20.2754) knots 0 0 0 1 2 2 2
  spline S133 degree 2 poles (-29.5871, 20.2754) (-29.7955, 19.9469) (-29.9189, 19.1183) (-29.8225, 18.6477) knots 0 0 0 1 2 2 2
  line L149 (-29.8225, 18.6477) -> (-26.3967, 16.4745)
  line L150 (-26.3967, 16.4745) -> (-26.9127, 15.6611)
  line L151 (-26.9127, 15.6611) -> (-31.7412, 18.7241)
  line L152 (-31.7412, 18.7241) -> (-31.2252, 19.5375)
  line L153 (-31.2252, 19.5375) -> (-30.5056, 19.081)
  spline S134 degree 2 poles (-30.5056, 19.081) (-30.6208, 19.7757) (-30.524, 20.643) (-30.3255, 20.9558) knots 0 0 0 1 2 2 2
  spline S135 degree 2 poles (-30.3255, 20.9558) (-30.2461, 21.081) (-30.1563, 21.1995) (-30.091, 21.2678) knots 0 0 0 1 2 2 2
  line L154 (-30.091, 21.2678) -> (-29.2463, 20.7319)
  line L155 (-24.1987, 19.5652) -> (-24.7927, 18.8069)
  line L156 (-24.7927, 18.8069) -> (-29.2943, 22.3327)
  line L157 (-29.2943, 22.3327) -> (-28.7003, 23.0911)
  line L158 (-28.7003, 23.0911) -> (-24.1987, 19.5652)
  line L159 (-29.4071, 23.731) -> (-30.081, 22.8705)
  line L160 (-30.081, 22.8705) -> (-30.8686, 23.4873)
  line L161 (-30.8686, 23.4873) -> (-30.1946, 24.3478)
  line L162 (-30.1946, 24.3478) -> (-29.4071, 23.731)
  spline S136 degree 2 poles (-22.0291, 26.1953) (-21.0266, 25.1719) (-20.8175, 23.0083) (-21.563, 22.278) knots 0 0 0 1 2 2 2
  spline S137 degree 2 poles (-21.563, 22.278) (-21.8674, 21.9799) (-22.4733, 21.663) (-22.8585, 21.5709) knots 0 0 0 1 2 2 2
  line L163 (-22.8585, 21.5709) -> (-21.1819, 19.8593)
  line L164 (-21.1819, 19.8593) -> (-21.8701, 19.1852)
  line L165 (-21.8701, 19.1852) -> (-27.3449, 24.7743)
  line L166 (-27.3449, 24.7743) -> (-26.6567, 25.4484)
  line L167 (-26.6567, 25.4484) -> (-26.2375, 25.0205)
  spline S138 degree 2 poles (-26.2375, 25.0205) (-26.2107, 25.505) (-25.8868, 26.4273) (-25.5206, 26.786) knots 0 0 0 1 2 2 2
  spline S139 degree 2 poles (-25.5206, 26.786) (-24.8192, 27.473) (-22.9451, 27.1305) (-22.0291, 26.1953) knots 0 0 0 1 2 2 2
  spline S140 degree 2 poles (-22.6615, 25.4202) (-23.3485, 26.1216) (-24.5503, 26.4572) (-25.0488, 25.9689) knots 0 0 0 1 2 2 2
  spline S141 degree 2 poles (-25.0488, 25.9689) (-25.3399, 25.6837) (-25.632, 24.8876) (-25.6758, 24.4471) knots 0 0 0 1 2 2 2
  line L168 (-25.6758, 24.4471) -> (-23.4029, 22.1267)
  spline S142 degree 2 poles (-23.4029, 22.1267) (-23.0085, 22.2624) (-22.5297, 22.5413) (-22.2826, 22.7832) knots 0 0 0 1 2 2 2
  spline S143 degree 2 poles (-22.2826, 22.7832) (-21.7489, 23.3061) (-21.9269, 24.6703) (-22.6615, 25.4202) knots 0 0 0 1 2 2 2
  spline S144 degree 2 poles (-16.8133, 29.6322) (-16.008, 28.4324) (-16.2841, 26.3507) (-17.2481, 25.7037) knots 0 0 0 1 2 2 2
  spline S145 degree 2 poles (-17.2481, 25.7037) (-18.2376, 25.0396) (-20.2758, 25.6275) (-21.0535, 26.7863) knots 0 0 0 1 2 2 2
  spline S146 degree 2 poles (-21.0535, 26.7863) (-21.8519, 27.9758) (-21.5673, 30.0781) (-20.6136, 30.7182) knots 0 0 0 1 2 2 2
  spline S147 degree 2 poles (-20.6136, 30.7182) (-19.6497, 31.3652) (-17.6151, 30.8269) (-16.8133, 29.6322) knots 0 0 0 1 2 2 2
  spline S148 degree 2 poles (-17.6388, 29.0782) (-18.2582, 30.0011) (-19.5321, 30.4475) (-20.1525, 30.0311) knots 0 0 0 1 2 2 2
  spline S149 degree 2 poles (-20.1525, 30.0311) (-20.7729, 29.6147) (-20.8475, 28.2632) (-20.228, 27.3403) knots 0 0 0 1 2 2 2
  spline S150 degree 2 poles (-20.228, 27.3403) (-19.6258, 26.4431) (-18.3296, 25.9744) (-17.7092, 26.3908) knots 0 0 0 1 2 2 2
  spline S151 degree 2 poles (-17.7092, 26.3908) (-17.0939, 26.8038) (-17.0262, 28.1655) (-17.6388, 29.0782) knots 0 0 0 1 2 2 2
  line L169 (-10.3034, 29.4417) -> (-11.1879, 29.0603)
  line L170 (-11.1879, 29.0603) -> (-11.4178, 29.5933)
  spline S152 degree 2 poles (-11.4178, 29.5933) (-11.5486, 29.3351) (-11.7513, 28.9787) (-11.9138, 28.7943) knots 0 0 0 1 2 2 2
  spline S153 degree 2 poles (-11.9138, 28.7943) (-12.0618, 28.6228) (-12.4228, 28.3528) (-12.6893, 28.2379) knots 0 0 0 1 2 2 2
  spline S154 degree 2 poles (-12.6893, 28.2379) (-13.1203, 28.052) (-14.0001, 28.0963) (-14.4044, 28.3321) knots 0 0 0 1 2 2 2
  spline S155 degree 2 poles (-14.4044, 28.3321) (-14.8088, 28.5679) (-15.5325, 29.4663) (-15.8186, 30.1297) knots 0 0 0 1 2 2 2
  spline S156 degree 2 poles (-15.8186, 30.1297) (-16.1169, 30.8215) (-16.195, 31.9848) (-16.0469, 32.4992) knots 0 0 0 1 2 2 2
  spline S157 degree 2 poles (-16.0469, 32.4992) (-15.9045, 32.9642) (-15.2624, 33.7051) (-14.8144, 33.8983) knots 0 0 0 1 2 2 2
  spline S158 degree 2 poles (-14.8144, 33.8983) (-14.4232, 34.067) (-13.7634, 34.1431) (-13.3619, 34.1011) knots 0 0 0 1 2 2 2
  line L171 (-13.3619, 34.1011) -> (-14.3401, 36.3691)
  line L172 (-14.3401, 36.3691) -> (-13.4555, 36.7506)
  line L173 (-13.4555, 36.7506) -> (-10.3034, 29.4417)
  line L174 (-11.7382, 30.336) -> (-13.0465, 33.3696)
  spline S159 degree 2 poles (-13.0465, 33.3696) (-13.4438, 33.3865) (-14.0168, 33.2806) (-14.3173, 33.151) knots 0 0 0 1 2 2 2
  spline S160 degree 2 poles (-14.3173, 33.151) (-14.9977, 32.8576) (-15.3287, 31.5044) (-14.913, 30.5404) knots 0 0 0 1 2 2 2
  spline S161 degree 2 poles (-14.913, 30.5404) (-14.512, 29.6105) (-13.4992, 28.8839) (-12.8471, 29.1651) knots 0 0 0 1 2 2 2
  spline S162 degree 2 poles (-12.8471, 29.1651) (-12.5012, 29.3143) (-11.9351, 29.9351) (-11.7382, 30.336) knots 0 0 0 1 2 2 2
  line L175 (-7.517, 30.1994) -> (-8.6975, 29.8811)
  line L176 (-8.6975, 29.8811) -> (-9.077, 31.2881)
  line L177 (-9.077, 31.2881) -> (-7.8965, 31.6064)
  line L178 (-7.8965, 31.6064) -> (-7.517, 30.1994)
  line L179 (-4.9112, 30.7287) -> (-5.8599, 30.562)
  line L180 (-5.8599, 30.562) -> (-6.8496, 36.1938)
  line L181 (-6.8496, 36.1938) -> (-5.9009, 36.3605)
  line L182 (-5.9009, 36.3605) -> (-4.9112, 30.7287)
  line L183 (-5.9986, 37.3089) -> (-7.0751, 37.1197)
  line L184 (-7.0751, 37.1197) -> (-7.2482, 38.105)
  line L185 (-7.2482, 38.105) -> (-6.1717, 38.2941)
  line L186 (-6.1717, 38.2941) -> (-5.9986, 37.3089)
  spline S163 degree 2 poles (1.1354, 34.208) (1.1965, 32.7767) (-0.0948, 31.028) (-1.1374, 30.9835) knots 0 0 0 1 2 2 2
  spline S164 degree 2 poles (-1.1374, 30.9835) (-1.5631, 30.9654) (-2.2255, 31.1349) (-2.5735, 31.324) knots 0 0 0 1 2 2 2
  line L187 (-2.5735, 31.324) -> (-2.4713, 28.9302)
  line L188 (-2.4713, 28.9302) -> (-3.4337, 28.8891)
  line L189 (-3.4337, 28.8891) -> (-3.7675, 36.7058)
  line L190 (-3.7675, 36.7058) -> (-2.8051, 36.7469)
  line L191 (-2.8051, 36.7469) -> (-2.7795, 36.1484)
  spline S165 degree 2 poles (-2.7795, 36.1484) (-2.4356, 36.4907) (-1.578, 36.96) (-1.066, 36.9818) knots 0 0 0 1 2 2 2
  spline S166 degree 2 poles (-1.066, 36.9818) (-0.085, 37.0237) (1.0795, 35.5159) (1.1354, 34.208) knots 0 0 0 1 2 2 2
  spline S167 degree 2 poles (0.1468, 34.0545) (0.1049, 35.0355) (-0.5643, 36.0885) (-1.2614, 36.0587) knots 0 0 0 1 2 2 2
  spline S168 degree 2 poles (-1.2614, 36.0587) (-1.6686, 36.0414) (-2.4181, 35.6447) (-2.7453, 35.3464) knots 0 0 0 1 2 2 2
  line L192 (-2.7453, 35.3464) -> (-2.6067, 32.1013)
  spline S169 degree 2 poles (-2.6067, 32.1013) (-2.2227, 31.9385) (-1.6802, 31.8257) (-1.3347, 31.8404) knots 0 0 0 1 2 2 2
  spline S170 degree 2 poles (-1.3347, 31.8404) (-0.5882, 31.8723) (0.1916, 33.0057) (0.1468, 34.0545) knots 0 0 0 1 2 2 2
  spline S171 degree 2 poles (3.9632, 30.7569) (3.1834, 30.8402) (2.4005, 31.8243) (2.5035, 32.7883) knots 0 0 0 1 2 2 2
  line L193 (2.5035, 32.7883) -> (2.84, 35.9382)
  line L194 (2.84, 35.9382) -> (2.1953, 36.0071)
  line L195 (2.1953, 36.0071) -> (2.28, 36.7991)
  line L196 (2.28, 36.7991) -> (2.9247, 36.7302)
  line L197 (2.9247, 36.7302) -> (3.0992, 38.3635)
  line L198 (3.0992, 38.3635) -> (4.057, 38.2612)
  line L199 (4.057, 38.2612) -> (3.8825, 36.6279)
  line L200 (3.8825, 36.6279) -> (5.6447, 36.4396)
  line L201 (5.6447, 36.4396) -> (5.5601, 35.6475)
  line L202 (5.5601, 35.6475) -> (3.7979, 35.8358)
  line L203 (3.7979, 35.8358) -> (3.5086, 33.1281)
  spline S172 degree 2 poles (3.5086, 33.1281) (3.4627, 32.6982) (3.4428, 32.2222) (3.5256, 32.0084) knots 0 0 0 1 2 2 2
  spline S173 degree 2 poles (3.5256, 32.0084) (3.5925, 31.8212) (3.9603, 31.6018) (4.2919, 31.5663) knots 0 0 0 1 2 2 2
  spline S174 degree 2 poles (4.2919, 31.5663) (4.5252, 31.5414) (4.9762, 31.636) (5.0791, 31.6685) knots 0 0 0 1 2 2 2
  line L204 (5.0791, 31.6685) -> (5.1343, 31.6626)
  line L205 (5.1343, 31.6626) -> (5.0425, 30.803)
  spline S175 degree 2 poles (5.0425, 30.803) (4.7644, 30.7582) (4.2026, 30.7313) (3.9632, 30.7569) knots 0 0 0 1 2 2 2
  spline S176 degree 2 poles (15.3764, 33.1447) (15.2022, 32.6824) (14.5592, 31.9745) (14.1556, 31.7966) knots 0 0 0 1 2 2 2
  spline S177 degree 2 poles (14.1556, 31.7966) (13.6486, 31.572) (12.5074, 31.5732) (11.7447, 31.8607) knots 0 0 0 1 2 2 2
  line L206 (11.7447, 31.8607) -> (10.9415, 32.1634)
  line L207 (10.9415, 32.1634) -> (9.9397, 29.5054)
  line L208 (9.9397, 29.5054) -> (8.992, 29.8626)
  line L209 (8.992, 29.8626) -> (11.6795, 36.9929)
  line L210 (11.6795, 36.9929) -> (13.4708, 36.3178)
  spline S178 degree 2 poles (13.4708, 36.3178) (14.1064, 36.0782) (14.9178, 35.5348) (15.1695, 35.1694) knots 0 0 0 1 2 2 2
  spline S179 degree 2 poles (15.1695, 35.1694) (15.4658, 34.7475) (15.6007, 33.7398) (15.3764, 33.1447) knots 0 0 0 1 2 2 2
  spline S180 degree 2 poles (14.3774, 33.4882) (14.5168, 33.858) (14.4673, 34.497) (14.2726, 34.7683) knots 0 0 0 1 2 2 2
  spline S181 degree 2 poles (14.2726, 34.7683) (14.1039, 35.0035) (13.5487, 35.3513) (13.1037, 35.519) knots 0 0 0 1 2 2 2
  line L211 (13.1037, 35.519) -> (12.3179, 35.8152)
  line L212 (12.3179, 35.8152) -> (11.2464, 32.9723)
  line L213 (11.2464, 32.9723) -> (11.8936, 32.7284)
  spline S182 degree 2 poles (11.8936, 32.7284) (12.4714, 32.5106) (13.2518, 32.4276) (13.5744, 32.5832) knots 0 0 0 1 2 2 2
  spline S183 degree 2 poles (13.5744, 32.5832) (13.8688, 32.7164) (14.2489, 33.1473) (14.3774, 33.4882) knots 0 0 0 1 2 2 2
  line L214 (23.0573, 31.2817) -> (16.8135, 26.1859)
  line L215 (16.8135, 26.1859) -> (15.8844, 26.7615)
  line L216 (15.8844, 26.7615) -> (17.6662, 34.6213)
  line L217 (17.6662, 34.6213) -> (18.5901, 34.049)
  line L218 (18.5901, 34.049) -> (17.0522, 27.5562)
  line L219 (17.0522, 27.5562) -> (22.1807, 31.8247)
  line L220 (22.1807, 31.8247) -> (23.0573, 31.2817)
  spline S184 degree 2 poles (25.5384, 23.9478) (24.1442, 22.4447) (21.9645, 21.8471) (21.0545, 22.6911) knots 0 0 0 1 2 2 2
  spline S185 degree 2 poles (21.0545, 22.6911) (20.1309, 23.5478) (20.5973, 25.785) (21.962, 27.2564) knots 0 0 0 1 2 2 2
  spline S186 degree 2 poles (21.962, 27.2564) (23.3646, 28.7686) (25.5359, 29.3571) (26.4504, 28.5089) knots 0 0 0 1 2 2 2
  spline S187 degree 2 poles (26.4504, 28.5089) (27.3695, 27.6565) (26.8905, 25.4056) (25.5384, 23.9478) knots 0 0 0 1 2 2 2
  spline S188 degree 2 poles (22.9996, 23.1357) (23.3645, 23.3111) (24.2445, 24.0783) (24.7778, 24.6533) knots 0 0 0 1 2 2 2
  spline S189 degree 2 poles (24.7778, 24.6533) (25.3111, 25.2282) (26.0058, 26.1589) (26.1571, 26.5491) knots 0 0 0 1 2 2 2
  spline S190 degree 2 poles (26.1571, 26.5491) (26.3085, 26.9393) (26.1875, 27.5989) (25.8752, 27.8886) knots 0 0 0 1 2 2 2
  spline S191 degree 2 poles (25.8752, 27.8886) (25.5628, 28.1784) (24.8869, 28.2578) (24.4962, 28.0727) knots 0 0 0 1 2 2 2
  spline S192 degree 2 poles (24.4962, 28.0727) (24.1185, 27.8925) (23.2307, 27.0988) (22.7226, 26.551) knots 0 0 0 1 2 2 2
  spline S193 degree 2 poles (22.7226, 26.551) (22.1767, 25.9624) (21.5185, 25.1074) (21.3507, 24.6904) knots 0 0 0 1 2 2 2
  spline S194 degree 2 poles (21.3507, 24.6904) (21.1906, 24.2999) (21.3038, 23.6137) (21.6298, 23.3114) knots 0 0 0 1 2 2 2
  spline S195 degree 2 poles (21.6298, 23.3114) (21.9376, 23.0258) (22.6135, 22.9464) (22.9996, 23.1357) knots 0 0 0 1 2 2 2
  spline S196 degree 2 poles (30.3482, 22.891) (30.1823, 23.1139) (29.7453, 23.4737) (29.5025, 23.6241) knots 0 0 0 1 2 2 2
  spline S197 degree 2 poles (29.5025, 23.6241) (29.2709, 23.7596) (28.875, 23.9191) (28.711, 23.9741) knots 0 0 0 1 2 2 2
  line L221 (28.711, 23.9741) -> (28.6741, 24.0236)
  line L222 (28.6741, 24.0236) -> (29.541, 24.6688)
  spline S198 degree 2 poles (29.541, 24.6688) (29.8838, 24.5081) (30.7986, 23.7649) (31.1046, 23.3537) knots 0 0 0 1 2 2 2
  spline S199 degree 2 poles (31.1046, 23.3537) (31.4142, 22.9376) (31.7066, 22.193) (31.7163, 21.8077) knots 0 0 0 1 2 2 2
  spline S200 degree 2 poles (31.7163, 21.8077) (31.7221, 21.3964) (31.3688, 20.7024) (30.9923, 20.4222) knots 0 0 0 1 2 2 2
  spline S201 degree 2 poles (30.9923, 20.4222) (30.487, 20.0462) (29.2301, 20.1424) (28.7845, 20.5343) knots 0 0 0 1 2 2 2
  line L223 (28.7845, 20.5343) -> (28.725, 20.4901)
  spline S202 degree 2 poles (28.725, 20.4901) (28.8292, 20.2674) (28.9789, 19.6938) (28.9406, 19.3728) knots 0 0 0 1 2 2 2
  spline S203 degree 2 poles (28.9406, 19.3728) (28.9073, 19.0555) (28.5294, 18.4049) (28.1282, 18.1063) knots 0 0 0 1 2 2 2
  spline S204 degree 2 poles (28.1282, 18.1063) (27.717, 17.8003) (26.8084, 17.5629) (26.3492, 17.6214) knots 0 0 0 1 2 2 2
  spline S205 degree 2 poles (26.3492, 17.6214) (25.8727, 17.6825) (25.0213, 18.2266) (24.6637, 18.7072) knots 0 0 0 1 2 2 2
  spline S206 degree 2 poles (24.6637, 18.7072) (24.3209, 19.1679) (23.8729, 20.2354) (23.7979, 20.6568) knots 0 0 0 1 2 2 2
  line L224 (23.7979, 20.6568) -> (24.6649, 21.3019)
  line L225 (24.6649, 21.3019) -> (24.7091, 21.2425)
  spline S207 degree 2 poles (24.7091, 21.2425) (24.7126, 20.8448) (25.0146, 19.7149) (25.3353, 19.2839) knots 0 0 0 1 2 2 2
  spline S208 degree 2 poles (25.3353, 19.2839) (25.5233, 19.0312) (26.0578, 18.6439) (26.3665, 18.6118) knots 0 0 0 1 2 2 2
  spline S209 degree 2 poles (26.3665, 18.6118) (26.6714, 18.5848) (27.2364, 18.7358) (27.5683, 18.9828) knots 0 0 0 1 2 2 2
  spline S210 degree 2 poles (27.5683, 18.9828) (27.9002, 19.2297) (28.1874, 19.7437) (28.1823, 20.0092) knots 0 0 0 1 2 2 2
  spline S211 degree 2 poles (28.1823, 20.0092) (28.1771, 20.2748) (27.921, 20.8154) (27.7146, 21.0928) knots 0 0 0 1 2 2 2
  line L226 (27.7146, 21.0928) -> (27.4565, 21.4396)
  line L227 (27.4565, 21.4396) -> (28.1352, 21.9447)
  line L228 (28.1352, 21.9447) -> (28.338, 21.6722)
  spline S212 degree 2 poles (28.338, 21.6722) (28.7472, 21.1223) (29.7884, 20.8195) (30.2887, 21.1918) knots 0 0 0 1 2 2 2
  spline S213 degree 2 poles (30.2887, 21.1918) (30.5216, 21.3651) (30.7208, 21.7904) (30.7129, 22.0078) knots 0 0 0 1 2 2 2
  spline S214 degree 2 poles (30.7129, 22.0078) (30.7027, 22.2388) (30.5067, 22.678) (30.3482, 22.891) knots 0 0 0 1 2 2 2
  dimension "d18" = 69.85
  constraints: 1 centre point, 1 coincident, 1 other
  measures "d18" diameter of A0
extrude "ExtrusionForText" cut sketch "Sketch5" against normal blind 1.27
sketch "Sketch13" plane through (0, -9.525, 0) normal (0, -1, 0) x (1, 0, 0)
  point P0 (0, 0)
  point P1 (44.45, 0)
  point P2 (22.225, 38.4948)
  point P3 (-22.225, 38.4948)
  point P4 (-44.45, 0)
  point P5 (-22.225, -38.4948)
  point P6 (22.225, -38.4948)
  dimension "d65" = 44.45
  dimension "d68" = 360
  constraints: 7 other
  measures "d65" distance of point (44.45, 0) point (0, 0)
hole "Hole6" at (44.45, -9.525, 0) at (22.225, -9.525, 38.4948) at (-22.225, -9.525, 38.4948) at (-44.45, -9.525, 0) at (-22.225, -9.525, -38.4948) at (22.225, -9.525, -38.4948) direction (0, 1, 0) diameter 6.3246 end through all counterbore diameter 6.5278 counterbore depth 6.1214
fillet "Fillet2" radius 1.27 1 edges at (10.795, -44.525, 0)
sketch "Sketch16" plane through (0, 0, 0) normal (0, 1, 0) x (1, 0, 0)
  point P0 (0, 0)
  point P1 (0, 0)
  constraints: 1 coincident
hole "Hole7" at (0, 0, 0) direction (0, -1, 0) diameter 11.9888 end through all clearance for "Flat Head Machine Screw" size "M10" standard "Ansi Metric M Profile"
sketch "Sketch18" plane through (0, 0, 0) normal (0, 1, 0) x (1, 0, 0)
  line L0 (9.9616, 0) -> (4.9808, -8.627)
  line L1 (4.9808, -8.627) -> (-4.9808, -8.627)
  line L2 (-4.9808, -8.627) -> (-9.9616, 0)
  line L3 (-9.9616, 0) -> (-4.9808, 8.627)
  line L4 (-4.9808, 8.627) -> (4.9808, 8.627)
  line L5 (4.9808, 8.627) -> (9.9616, 0)
  point P0 (0, 0)
  point P1 (0, 0)
  dimension "d104" = 17.254
  constraints: 12 end point, 1 coincident, 1 horizontal, 13 other
  measures "d104" distance between parallel lines of L1 L4
extrude "Extrusion8" cut sketch "Sketch18" against normal blind 33.4
equation "\"d18\" = textDiameter"
equation "\"d0\" = topRadius"
equation "\"d3\" = topThickness"
equation "\"d4\" = depthIntoTripod"
equation "\"depthIntoTripod\" = 35"
equation "\"insertionPointDiameter\" = 25.4"
equation "\"topDiameter\" = 120.65"
equation "\"topRadius\" = 0.5 * topDiameter"
equation "\"topThickness\" = 9.525"
equation "\"hexBoltClearance\" = 17.635"
equation "\"totalPartHeight\" = depthIntoTripod + topThickness"
equation "\"hexBoltDepth\" = totalPartHeight - hexBoltSupport"
equation "\"hexBoltSupport\" = 9.525"
equation "\"holeForGearBoxHardware\" = 50.8"
equation "\"depthForGearBoxHardware\" = 6.35"
equation "\"textDiameter\" = 69.85"
body "Solid1"
